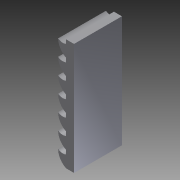
# Autodesk Inventor part: ratchet
Saved by Autodesk Inventor 2012 (Build 160160000, 160)
## iProperties
Created: 2012-01-29
Part Number: ratchet
Material: Default
Document SubType Name: Modeling
Designer: Antonella Wilby
Density: 1 g/cm^3
Author: Antonella Wilby
Autodesk Inventor part; units mm, degrees
ref_plane "YZ Plane" through (0, 0, 0) normal (1, 0, 0) x (0, 1, 0)
ref_plane "XZ Plane" through (0, 0, 0) normal (0, 1, 0) x (-1, 0, 0)
ref_plane "XY Plane" through (0, 0, 0) normal (0, 0, 1) x (1, 0, 0)
sketch "Sketch1" plane through (0, 0, 0) normal (0, 0, 1) x (1, 0, 0)
  line L0 (-3.81, 0) -> (0.635, 0) projected
  line L1 (0, -31.115) -> (0, 31.115) projected
  line L2 (0, -22.225) -> (0, 22.225)
  line L3 (0, -22.225) -> (-3.175, -22.225)
  line L4 (0, 22.225) -> (-3.175, 22.225)
  line L5 (-3.175, 22.225) -> (-3.175, -22.225) construction
  line L6 (-3.175, -22.225) -> (-3.175, 22.225)
  point P0 (0, 0)
  point P1 (0, 0)
  point P2 (-3.175, -18.1789)
  dimension "d0" = 44.45
  dimension "d3" = 3.175
  constraints: 10 end point, 4 point on line, 2 equal length, 2 perpendicular, 1 coincident, 1 midpoint
  measures "d0" distance of L2.start L2.end
  measures "d3" distance of L2.start L3.end
extrude "Extrusion1" add sketch "Sketch1" along normal mid plane 19.05
sketch "Sketch2" plane through (0, 0, 0) normal (0, 0, 1) x (1, 0, 0)
  line L0 (-3.175, -22.225) -> (-3.175, 22.225) projected
  line L1 (0, -22.225) -> (-3.175, -22.225) projected
  line L2 (0, 22.225) -> (0, -22.225) projected
  line L3 (-3.175, 22.225) -> (0, 22.225) projected
  line L4 (-6.35, -22.225) -> (-6.35, 22.225) construction
  arc A0 (-6.35, -17.145) -> (-3.175, -22.225) centre (-0.6351, -17.1054) ccw
  arc A1 (-6.35, -17.145) -> (-3.175, -17.4625) centre (-4.4894, -14.5723) ccw
  line L5 (-6.35, -17.145) -> (0, -17.145) construction
  point P0 (0, 0)
  dimension "d10" = 3.175
  dimension "d11" = 5.08
  dimension "d12" = 5.715
  dimension "d14" = 3.175
  dimension "d15" = 0.3175
  constraints: 4 end point, 4 point on circle, 3 point on line, 2 centre point, 2 perpendicular
  measures "d10" distance between parallel lines of L4 L0
  measures "d11" distance between parallel lines of L5 L1
  measures "d12" radius of A0
  measures "d14" radius of A1
  measures "d15" distance from line of L5 A1.end
extrude "Extrusion2" add sketch "Sketch2" along normal mid plane 19.05 contours A0 A1 L0
pattern_linear "Rectangular Pattern1" count 7 spacing 6.35 along (0, 1, 0) of "Extrusion2"
body "Solid1"
